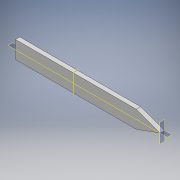
# Autodesk Inventor part: socket_pin
Saved by Autodesk Inventor 2018 (Build 220112000, 112)
## iProperties
Created: 2017-04-13
Part Number: socket_pin
Material: Generic
Document SubType Name: Modeling
Designer: kampe_000
Density: 1 g/cm^3
Appearance: Default
Author: kampe_000
Autodesk Inventor part; units mm, degrees
ref_plane "YZ Plane" through (0, 0, 0) normal (1, 0, 0) x (0, 1, 0)
ref_plane "XZ Plane" through (0, 0, 0) normal (0, 1, 0) x (-1, 0, 0)
ref_plane "XY Plane" through (0, 0, 0) normal (0, 0, 1) x (1, 0, 0)
sketch "Sketch1" plane through (0, 0, 0) normal (0, 1, 0) x (-1, 0, 0)
  line L0 (0, 0) -> (-4.1758, 0)
  line L1 (-4.1758, 0) -> (-5, -0.3)
  line L2 (-5, -0.3) -> (-4.1758, -0.6)
  line L3 (-4.1758, -0.6) -> (0, -0.6)
  line L4 (0, -0.6) -> (0, 0)
  line L5 (0, -0.3) -> (-15.0244, -0.3) construction
  dimension "d0" = 0.6
  dimension "d1" = 160
  dimension "d2" = 160
  dimension "d3" = 5
  constraints: 12 end point, 2 horizontal, 1 midpoint, 1 parallel, 1 perpendicular, 1 point on line
  measures "d0" distance of L3.end L0.start
  measures "d1" angle of L3 L2
  measures "d2" angle of L1 L0
  measures "d3" distance from line of L4 L1.end
extrude "Extrusion1" add sketch "Sketch1" along normal blind 0.15
ref_plane "pinLenght" through (2, 0, -0.3) normal (-1, 0, 0) x (0, 1, 0)
ref_plane "Work Plane2" through (5, 0, -0.3) normal (-1, 0, 0) x (0, 1, 0)
ref_plane "Work Plane1" through (4.1758, 0, -0.3) normal (0, 0, -1) x (-1, 0, 0)
equation "\"d2\" = d1"
body "Solid1"
